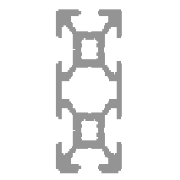
# Autodesk Inventor part: 3 842 992 891-0mm
Saved by Autodesk Inventor 2023.2 (Build 272271000, 271)
## iProperties
RuleStatus: InUse
Created: 2023-01-25
Part Number: 3 842 992 891-0mm
Material: Aluminum-6061
Description: PROFILE 20x40
Document SubType Name: Modeling
Designer: dmargari
Manufacturer: GENERIC
Standards Organization: ISO
Language: en-US
Size Designation: 300
Categories: <MemberInstance><Categories><Category DisplayName="Structural Shapes" InternalName="089c4875-fa83-4c05-b084-43b9cc11f5ed" Mnemonic="GRDR"><CategoryParameter DisplayName="Mass per Length Unit" InternalName="0bb95a10-148f-4027-a459-38d7b056702a" Mnemonic="shpmass"/><CategoryParameter DisplayName="Section Area" InternalName="1ff91680-64b0-4202-b9a3-7fd3f94bba3b" Mnemonic="secarea"/><CategoryParameter DisplayName="Radius of Gyration (x)" InternalName="25778675-03e9-40c1-b6a8-4a9ed693320d" Mnemonic="gyrradx"/><CategoryParameter DisplayName="Torsional Rigidity Modulus" InternalName="26c1ec35-5026-4c63-ad0a-751cf684a536" Mnemonic="torrigmod"/><CategoryParameter DisplayName="Distance of the Center of Gravity X-X" InternalName="26c9bdb8-9c79-4b4f-a92e-8e197583c9c4" Mnemonic="grcendistX"/><CategoryParameter DisplayName="Legacy Member ID" InternalName="340afe4f-75d7-48d3-ab7d-943f3c3da468" Mnemonic="LegacyMemberID"/><CategoryParameter DisplayName="Base Length" InternalName="42e34263-8f20-4d0e-ad48-bf1385b87c24" Mnemonic="shplen"/><CategoryParameter DisplayName="Moment of Inertia (y)" InternalName="4b9f58ea-bced-460e-81ea-3d29ca5a49e3" Mnemonic="inermomy"/><CategoryParameter DisplayName="Moment of Inertia (x)" InternalName="4cd780bc-73d7-43ac-917a-579e5cbd684d" Mnemonic="inermomx"/><CategoryParameter DisplayName="Custom Base Point" InternalName="4f1d1b73-316d-484b-a3df-9cbabb16eb77" Mnemonic="shpBasePoint"/><CategoryParameter DisplayName="Shape Height" InternalName="50274e7d-5ac0-4796-92cb-c59e54983c67" Mnemonic="shpheig"/><CategoryParameter DisplayName="Section Module (y)" InternalName="59eaa5e9-d227-48dc-b6c1-6920f96e0f95" Mnemonic="secmody"/><CategoryParameter DisplayName="Section Designation" InternalName="5a64d034-428d-49c8-ba32-7619764de20f" Mnemonic="shpdes"/><CategoryParameter DisplayName="Section Module (x)" InternalName="72cfad18-cf51-4ed4-aaa7-c6b224f8419f" Mnemonic="secmodx"/><CategoryParameter DisplayName="Torsional Section Modulus" InternalName="7c55a8dc-8844-49f9-a867-cc677b30ec9a" Mnemonic="torsecmod"/><CategoryParameter DisplayName="Shape Width" InternalName="7c717d54-a18f-4666-b4d4-573cce22c62c" Mnemonic="shpwdth"/><CategoryParameter DisplayName="Second Shape Thickness" InternalName="9251a8e1-85fd-4e47-af99-afdb762317d9" Mnemonic="shpthick2"/><CategoryParameter DisplayName="FG Authored" InternalName="9c666724-f362-4ea7-ac62-f6a007de5c69" Mnemonic="shpFGAuto"/><CategoryParameter DisplayName="Distance of the Center of Gravity Y-Y" InternalName="bcc4fb17-7af4-436a-8f8c-d0aa3b0248c5" Mnemonic="grcendistY"/><CategoryParameter DisplayName="Radius of Gyration (y)" InternalName="bfa18ebe-1636-4dbe-8d42-b263e0b73184" Mnemonic="gyrrady"/><CategoryParameter DisplayName="Shape Thickness" InternalName="d109cf76-8eb4-42fc-9800-4409734adc67" Mnemonic="shpthick"/><CategoryParameter DisplayName="Coefficient of Shear Displacement" InternalName="de4c90c6-aaa8-468f-a335-6737b311b5d3" Mnemonic="shdispc"/><Category DisplayName="Other" InternalName="f02205ff-2390-476f-921c-0b3185f88e84" Mnemonic="OTHSHP"><CategoryParameter DisplayName="Moment of Inertia (y)" InternalName="044c654e-f649-48ac-84cc-650a29ae31ca" Mnemonic="inermomy"/><CategoryParameter DisplayName="Shape Thickness" InternalName="12b1a788-9233-48fd-a933-2df8ff42b15f" Mnemonic="shpthick"/><CategoryParameter DisplayName="Mass per Length Unit" InternalName="2fd289d6-9394-4d2d-97e6-6659d7d4551d" Mnemonic="shpmass"/><CategoryParameter DisplayName="Radius of Gyration (y)" InternalName="743e1dfe-1bba-408b-b985-cf752b207386" Mnemonic="gyrrady"/><CategoryParameter DisplayName="Section Module (y)" InternalName="88b8bff9-a616-4028-93d5-ed4f79680d13" Mnemonic="secmody"/><CategoryParameter DisplayName="Section Area" InternalName="c46ecdf8-b6eb-4db9-8b25-30258930c1e3" Mnemonic="secarea"/><CategoryParameter DisplayName="Section Module (x)" InternalName="cac70804-9d39-43bb-be17-56ea1f39a6c2" Mnemonic="secmodx"/><CategoryParameter DisplayName="Moment of Inertia (x)" InternalName="ec6737bc-264f-43ed-b0bd-f6d410c2718d" Mnemonic="inermomx"/><CategoryParameter DisplayName="Radius of Gyration (x)" InternalName="ee72c61e-565e-4fd6-b448-66e1e1abcb7e" Mnemonic="gyrradx"/></Category></Category><Category DisplayName="DataType" InternalName="23b78d0f-2648-40c6-8793-ca6db495c9e8" Mnemonic="DATATYPE"><CategoryParameter DisplayName="DisplayName" InternalName="05415f3d-3907-474b-a020-eb9d644f4cf3" Mnemonic="DISPLAYNAME"/><CategoryParameter DisplayName="Standard" InternalName="0c0a119c-1e12-4c84-803f-101930972f5e" Mnemonic="STANDARD"/><CategoryParameter DisplayName="Description" InternalName="13903e3d-64b1-4950-80da-f627842ea37f" Mnemonic="DESCRIPTION"/><CategoryParameter DisplayName="Designation" InternalName="2675968c-4ce5-49e0-a4f5-552d29089031" Mnemonic="DESIGNATION"/><CategoryParameter DisplayName="Default Row" InternalName="2af9ec52-faaa-4026-b378-f9fa4afca842" Mnemonic="DEFAULTROW"/><CategoryParameter DisplayName="Folder Name" InternalName="3f06958e-8713-4116-9be7-ed6184ecc97b" Mnemonic="FOLDERNAME"/><CategoryParameter DisplayName="Revision Guid" InternalName="45a75005-10b1-4dfc-8d6d-dfe629f0b93c" Mnemonic="REVISIONGUID"/><CategoryParameter DisplayName="FileName" InternalName="8b46a4cc-9585-4fed-90c3-899f57e09a73" Mnemonic="FILENAME"/><CategoryParameter DisplayName="StdsOrg" InternalName="8f5914e1-4693-403f-8ab5-d37768198c9d" Mnemonic="STDSORG"/><CategoryParameter DisplayName="Family Version" InternalName="914462f6-6e19-4b14-ba84-155b9680b1d0" Mnemonic="FAMILYREVISION"/><CategoryParameter DisplayName="Standard Revision" InternalName="91d5a463-65c2-4fde-b823-3b7fea5e8e17" Mnemonic="STANDARDREVISION"/><CategoryParameter DisplayName="Member Revision" InternalName="a65d44b9-392f-4f4f-857b-e4b3d54996fe" Mnemonic="MEMBERREVISION"/><CategoryParameter DisplayName="ClipFormat" InternalName="bc51e27b-3422-4e78-93ef-cec197ddf230" Mnemonic="CLIPFORMAT"/><CategoryParameter DisplayName="Manufacturer" InternalName="cd6c7a72-a28a-4e50-99a9-2c7f4e13e5ad" Mnemonic="MANUFACTURER"/><CategoryParameter DisplayName="InternalName" InternalName="cf1d0246-76d9-4b4a-8305-fa0409afb5c1" Mnemonic="INTERNALNAME"/><CategoryParameter DisplayName="IsMetric" InternalName="e2385c5b-1ea4-4823-96a8-8de651266ec3" Mnemonic="ISMETRIC"/><Category DisplayName="Part" InternalName="c0e0b642-3bcb-4cc8-9e80-f96d35c4afa4" Mnemonic="PART"><CategoryParameter DisplayName="Part Number" InternalName="016b6077-bfbe-49bd-92c9-d8d59c39c941" Mnemonic="PARTNUMBER"/><CategoryParameter DisplayName="Stock Number" InternalName="4dba7c1c-e26c-444e-836c-b08b433409a8" Mnemonic="STOCKNUMBER"/><CategoryParameter DisplayName="Material Key" InternalName="5c9a8adb-dd2b-4535-b97f-0a94a95fe41f" Mnemonic="MATERIALKEY"/><CategoryParameter DisplayName="Material" InternalName="818a152a-d3c3-49ca-80ee-df7d91421b8e" Mnemonic="MATERIAL"/></Category></Category></Categories><FamilyTemplate Id="20x40"><FamilyTemplateParameters><FamilyTemplateParameter ObjectType="kModelParameterObject" ValueType="xs:double" Id="12" ObjectReferenceKey="Length"/><FamilyTemplateParameter ObjectType="kPartComponentDefinitionObject" ValueType="xs:string" Id="23" SubObjectId="Material"/><FamilyTemplateParameter ObjectType="kPropertyObject" ValueType="xs:string" Id="26" ObjectReferenceKey="{32853F0F-3444-11d1-9E93-0060B03C1CA6}" SubObjectId="5"/><FamilyTemplateParameter ObjectType="kPropertyObject" ValueType="xs:string" Id="27" ObjectReferenceKey="{32853F0F-3444-11d1-9E93-0060B03C1CA6}" SubObjectId="52"/></FamilyTemplateParameters></FamilyTemplate><CategoryParameterMap><ParamToTemplateMap><ParamToTemplate CategoryParameter="//CategoryParameter[@InternalName='cf1d0246-76d9-4b4a-8305-fa0409afb5c1']" ConstantValue="b55e8ed9-29f0-457f-be10-b8c2b92fdd42"/><ParamToTemplate CategoryParameter="//CategoryParameter[@InternalName='45a75005-10b1-4dfc-8d6d-dfe629f0b93c']" ConstantValue="8c683705-cc53-472d-bb0d-51e7db6332bf"/><ParamToTemplate CategoryParameter="//CategoryParameter[@InternalName='3f06958e-8713-4116-9be7-ed6184ecc97b']" ConstantValue="20x40"/><ParamToTemplate CategoryParameter="//CategoryParameter[@InternalName='8f5914e1-4693-403f-8ab5-d37768198c9d']" ConstantValue="ISO"/><ParamToTemplate CategoryParameter="//CategoryParameter[@InternalName='0c0a119c-1e12-4c84-803f-101930972f5e']" TemplateParameter="18"/><ParamToTemplate CategoryParameter="//CategoryParameter[@InternalName='91d5a463-65c2-4fde-b823-3b7fea5e8e17']" TemplateParameter="19"/><ParamToTemplate CategoryParameter="//CategoryParameter[@InternalName='cd6c7a72-a28a-4e50-99a9-2c7f4e13e5ad']" ConstantValue="GENERIC"/><ParamToTemplate CategoryParameter="//CategoryParameter[@InternalName='13903e3d-64b1-4950-80da-f627842ea37f']" ConstantValue="PROFILE 20x40"/><ParamToTemplate CategoryParameter="//CategoryParameter[@InternalName='05415f3d-3907-474b-a020-eb9d644f4cf3']" ConstantValue="20x40"/><ParamToTemplate CategoryParameter="//CategoryParameter[@InternalName='914462f6-6e19-4b14-ba84-155b9680b1d0']" ConstantValue="11"/><ParamToTemplate CategoryParameter="//CategoryParameter[@InternalName='bc51e27b-3422-4e78-93ef-cec197ddf230']" ConstantValue="CF_INVENTOR.STDPARTS"/><ParamToTemplate CategoryParameter="//CategoryParameter[@InternalName='e2385c5b-1ea4-4823-96a8-8de651266ec3']" ConstantValue="true"/><ParamToTemplate CategoryParameter="//CategoryParameter[@InternalName='2af9ec52-faaa-4026-b378-f9fa4afca842']" ConstantValue="1"/><ParamToTemplate CategoryParameter="//CategoryParameter[@InternalName='9c666724-f362-4ea7-ac62-f6a007de5c69']" ConstantValue="1"/><ParamToTemplate CategoryParameter="//CategoryParameter[@InternalName='8b46a4cc-9585-4fed-90c3-899f57e09a73']" ConstantValue="300"/><ParamToTemplate CategoryParameter="//CategoryParameter[@InternalName='a65d44b9-392f-4f4f-857b-e4b3d54996fe']" ConstantValue="6f428d9a-a522-4f2d-9c06-86253ee4d95b"/><ParamToTemplate CategoryParameter="//CategoryParameter[@InternalName='a65d44b9-392f-4f4f-857b-e4b3d54996fe']" ConstantValue="6f428d9a-a522-4f2d-9c06-86253ee4d95b"/><ParamToTemplate CategoryParameter="//CategoryParameter[@InternalName='2675968c-4ce5-49e0-a4f5-552d29089031']" TemplateParameter="27"/><ParamToTemplate CategoryParameter="//CategoryParameter[@InternalName='42e34263-8f20-4d0e-ad48-bf1385b87c24']" TemplateParameter="12"/><ParamToTemplate CategoryParameter="//CategoryParameter[@InternalName='818a152a-d3c3-49ca-80ee-df7d91421b8e']" TemplateParameter="23"/><ParamToTemplate CategoryParameter="//CategoryParameter[@InternalName='016b6077-bfbe-49bd-92c9-d8d59c39c941']" TemplateParameter="26"/></ParamToTemplateMap></CategoryParameterMap></MemberInstance>
Stock Number: 3 842 992 891
Mass: 1.55822 g
Surface Area: 12.24 cm^2
Volume: 0.57499 cm^3
Density: 2.71 g/cm^3
Appearance: Aluminum - Flat-1
IsCustomPart: 1
G_L: 300.000 mm
Author: dmargari
Autodesk Inventor part; units mm, degrees
(part 1 of 2)
ref_plane "YZ Plane" through (0, 0, 0) normal (1, 0, 0) x (0, 1, 0)
ref_plane "XZ Plane" through (0, 0, 0) normal (0, 1, 0) x (-1, 0, 0)
sketch "20x40" plane through (0, 0, 0) normal (0, 0, 1) x (1, 0, 0)
  line L0 (125.1239, 22.9032) -> (127.4025, 22.9032)
  arc A0 (127.5025, 22.8764) -> (127.4025, 22.9032) centre (127.4025, 22.7032) ccw
  line L1 (127.5025, 22.8764) -> (128.2563, 22.4412)
  arc A1 (128.2563, 22.4412) -> (128.4563, 22.4412) centre (128.3563, 22.6144) ccw
  line L2 (128.4563, 22.4412) -> (129.2101, 22.8764)
  arc A2 (129.3101, 22.9032) -> (129.2101, 22.8764) centre (129.3101, 22.7032) ccw
  line L3 (129.3101, 22.9032) -> (131.5887, 22.9032)
  arc A3 (131.5887, 22.9032) -> (131.9423, 23.0497) centre (131.5887, 23.4032) ccw
  line L4 (131.9423, 23.0497) -> (134.6492, 25.7567)
  arc A4 (135.0028, 25.9031) -> (134.6492, 25.7567) centre (135.0028, 25.4031) ccw
  line L5 (135.0028, 25.9031) -> (136.3563, 25.9031)
  arc A5 (136.3563, 25.9031) -> (136.8563, 26.4031) centre (136.3563, 26.4031) ccw
  line L6 (136.8563, 26.4031) -> (136.8563, 30.4031)
  arc A6 (136.8563, 30.4031) -> (136.3563, 30.9031) centre (136.3563, 30.4031) ccw
  line L7 (136.3563, 30.9031) -> (135.0028, 30.9031)
  arc A7 (134.6492, 31.0496) -> (135.0028, 30.9031) centre (135.0028, 31.4031) ccw
  line L8 (134.6492, 31.0496) -> (131.9421, 33.7567)
  arc A8 (131.9421, 33.7567) -> (131.5886, 33.9031) centre (131.5886, 33.4031) ccw
  line L9 (131.5886, 33.9031) -> (129.3099, 33.9031)
  arc A9 (129.2099, 33.9299) -> (129.3099, 33.9031) centre (129.3099, 34.1031) ccw
  line L10 (129.2099, 33.9299) -> (128.4563, 34.365)
  arc A10 (128.4563, 34.365) -> (128.2563, 34.365) centre (128.3563, 34.1918) ccw
  line L11 (128.2563, 34.365) -> (127.5027, 33.9299)
  arc A11 (134.2099, 45.3173) -> (134.3563, 45.6709) centre (133.8563, 45.6709) ccw
  line L12 (134.3563, 46.4031) -> (134.3563, 45.6709)
  arc A12 (134.3563, 46.4031) -> (133.8563, 46.9031) centre (133.8563, 46.4031) ccw
  line L13 (131.8563, 46.9031) -> (133.8563, 46.9031)
  arc A13 (131.3563, 47.4031) -> (131.8563, 46.9031) centre (131.8563, 47.4031) ccw
  line L14 (131.3563, 47.7031) -> (131.3563, 47.4031)
  arc A14 (131.5563, 47.9031) -> (131.3563, 47.7031) centre (131.5563, 47.7031) ccw
  line L15 (131.6563, 47.9031) -> (131.5563, 47.9031)
  arc A15 (131.6563, 47.9031) -> (131.8563, 48.1031) centre (131.6563, 48.1031) ccw
  line L16 (131.8563, 48.2031) -> (131.8563, 48.1031)
  arc A16 (132.0563, 48.4031) -> (131.8563, 48.2031) centre (132.0563, 48.2031) ccw
  line L17 (136.8563, 48.4031) -> (132.0563, 48.4031)
  arc A17 (138.3563, 46.9031) -> (136.8563, 48.4031) centre (136.8563, 46.9031) ccw
  line L18 (138.3563, 42.1031) -> (138.3563, 46.9031)
  arc A18 (138.1563, 41.9031) -> (138.3563, 42.1031) centre (138.1563, 42.1031) ccw
  line L19 (138.0563, 41.9031) -> (138.1563, 41.9031)
  arc A19 (138.0563, 41.9031) -> (137.8563, 41.7031) centre (138.0563, 41.7031) ccw
  line L20 (137.8563, 41.6031) -> (137.8563, 41.7031)
  arc A20 (137.6563, 41.4031) -> (137.8563, 41.6031) centre (137.6563, 41.6031) ccw
  line L21 (137.3563, 41.4031) -> (137.6563, 41.4031)
  arc A21 (136.8563, 41.9031) -> (137.3563, 41.4031) centre (137.3563, 41.9031) ccw
  line L22 (136.8563, 43.9031) -> (136.8563, 41.9031)
  arc A22 (136.8563, 43.9031) -> (136.3563, 44.4031) centre (136.3563, 43.9031) ccw
  line L23 (135.6241, 44.4031) -> (136.3563, 44.4031)
  arc A23 (135.6241, 44.4031) -> (135.2705, 44.2567) centre (135.6241, 43.9031) ccw
  line L24 (133.0028, 41.9889) -> (135.2705, 44.2567)
  arc A24 (133.0028, 41.9889) -> (132.8563, 41.6353) centre (133.3563, 41.6353) ccw
  line L25 (132.8563, 39.3567) -> (132.8563, 41.6353)
  arc A25 (132.8295, 39.2567) -> (132.8563, 39.3567) centre (132.6563, 39.3567) ccw
  line L26 (132.3944, 38.5031) -> (132.8295, 39.2567)
  arc A26 (132.3944, 38.5031) -> (132.3944, 38.3031) centre (132.5676, 38.4031) ccw
  line L27 (132.8295, 37.5495) -> (132.3944, 38.3031)
  arc A27 (132.8563, 37.4495) -> (132.8295, 37.5495) centre (132.6563, 37.4495) ccw
  line L28 (132.8563, 35.1709) -> (132.8563, 37.4495)
  arc A28 (132.8563, 35.1709) -> (133.0028, 34.8173) centre (133.3563, 35.1709) ccw
  line L29 (135.2705, 32.5496) -> (133.0028, 34.8173)
  arc A29 (135.2705, 32.5496) -> (135.6241, 32.4031) centre (135.6241, 32.9031) ccw
  line L30 (136.3563, 32.4031) -> (135.6241, 32.4031)
  arc A30 (136.3563, 32.4031) -> (136.8563, 32.9031) centre (136.3563, 32.9031) ccw
  line L31 (136.8563, 34.9031) -> (136.8563, 32.9031)
  arc A31 (137.3563, 35.4031) -> (136.8563, 34.9031) centre (137.3563, 34.9031) ccw
  line L32 (137.6563, 35.4031) -> (137.3563, 35.4031)
  arc A32 (137.8563, 35.2031) -> (137.6563, 35.4031) centre (137.6563, 35.2031) ccw
  line L33 (137.8563, 35.1031) -> (137.8563, 35.2031)
  arc A33 (137.8563, 35.1031) -> (138.0563, 34.9031) centre (138.0563, 35.1031) ccw
  line L34 (138.1563, 34.9031) -> (138.0563, 34.9031)
  arc A34 (138.3563, 34.7031) -> (138.1563, 34.9031) centre (138.1563, 34.7031) ccw
  line L35 (138.3563, 22.0531) -> (138.3563, 34.7031)
  arc A35 (138.1563, 21.8531) -> (138.3563, 22.0531) centre (138.1563, 22.0531) ccw
  line L36 (138.0563, 21.8531) -> (138.1563, 21.8531)
  arc A36 (138.0563, 21.8531) -> (137.8563, 21.6531) centre (138.0563, 21.6531) ccw
  line L37 (137.8563, 21.5531) -> (137.8563, 21.6531)
  arc A37 (137.6563, 21.3531) -> (137.8563, 21.5531) centre (137.6563, 21.5531) ccw
  line L38 (137.3563, 21.3531) -> (137.6563, 21.3531)
  arc A38 (136.8563, 21.8531) -> (137.3563, 21.3531) centre (137.3563, 21.8531) ccw
  line L39 (136.8563, 23.9031) -> (136.8563, 21.8531)
  arc A39 (136.8563, 23.9031) -> (136.3563, 24.4031) centre (136.3563, 23.9031) ccw
  line L40 (135.6241, 24.4031) -> (136.3563, 24.4031)
  arc A40 (135.6241, 24.4031) -> (135.2705, 24.2567) centre (135.6241, 23.9031) ccw
  line L41 (133.0028, 21.9889) -> (135.2705, 24.2567)
  arc A41 (133.0028, 21.9889) -> (132.8563, 21.6353) centre (133.3563, 21.6353) ccw
  line L42 (132.8563, 19.3567) -> (132.8563, 21.6353)
  arc A42 (132.8295, 19.2567) -> (132.8563, 19.3567) centre (132.6563, 19.3567) ccw
  line L43 (132.3944, 18.5031) -> (132.8295, 19.2567)
  arc A43 (132.3944, 18.5031) -> (132.3944, 18.3031) centre (132.5676, 18.4031) ccw
  line L44 (132.8295, 17.5495) -> (132.3944, 18.3031)
  arc A44 (132.8563, 17.4495) -> (132.8295, 17.5495) centre (132.6563, 17.4495) ccw
  line L45 (132.8563, 15.1709) -> (132.8563, 17.4495)
  arc A45 (132.8563, 15.1709) -> (133.0028, 14.8173) centre (133.3563, 15.1709) ccw
  line L46 (135.2705, 12.5496) -> (133.0028, 14.8173)
  arc A46 (135.2705, 12.5496) -> (135.6241, 12.4031) centre (135.6241, 12.9031) ccw
  line L47 (136.3563, 12.4031) -> (135.6241, 12.4031)
  arc A47 (136.3563, 12.4031) -> (136.8563, 12.9031) centre (136.3563, 12.9031) ccw
  line L48 (136.8563, 14.8531) -> (136.8563, 12.9031)
  arc A48 (137.3563, 15.3531) -> (136.8563, 14.8531) centre (137.3563, 14.8531) ccw
  line L49 (137.6563, 15.3531) -> (137.3563, 15.3531)
  arc A49 (137.8563, 15.1531) -> (137.6563, 15.3531) centre (137.6563, 15.1531) ccw
  line L50 (137.8563, 15.0531) -> (137.8563, 15.1531)
  arc A50 (137.8563, 15.0531) -> (138.0563, 14.8531) centre (138.0563, 15.0531) ccw
  line L51 (138.1563, 14.8531) -> (138.0563, 14.8531)
  arc A51 (138.3563, 14.6531) -> (138.1563, 14.8531) centre (138.1563, 14.6531) ccw
  arc A52 (127.4027, 33.9031) -> (127.5027, 33.9299) centre (127.4027, 34.1031) ccw
  line L52 (127.4027, 33.9031) -> (125.1241, 33.9031)
  arc A53 (125.1241, 33.9031) -> (124.7705, 33.7567) centre (125.1241, 33.4031) ccw
  line L53 (124.7705, 33.7567) -> (122.0634, 31.0496)
  arc A54 (121.7099, 30.9031) -> (122.0634, 31.0496) centre (121.7099, 31.4031) ccw
  line L54 (121.7099, 30.9031) -> (120.3563, 30.9031)
  arc A55 (120.3563, 30.9031) -> (119.8563, 30.4031) centre (120.3563, 30.4031) ccw
  line L55 (119.8563, 30.4031) -> (119.8563, 26.4031)
  arc A56 (119.8563, 26.4031) -> (120.3563, 25.9031) centre (120.3563, 26.4031) ccw
  line L56 (120.3563, 25.9031) -> (121.7099, 25.9031)
  arc A57 (122.0634, 25.7567) -> (121.7099, 25.9031) centre (121.7099, 25.4031) ccw
  line L57 (122.0634, 25.7567) -> (124.7703, 23.0497)
  arc A58 (124.7703, 23.0497) -> (125.1239, 22.9032) centre (125.1239, 23.4032) ccw
  arc A59 (118.3563, 9.9031) -> (119.8563, 8.4031) centre (119.8563, 9.9031) ccw
  line L58 (118.3563, 14.6531) -> (118.3563, 9.9031)
  arc A60 (118.5563, 14.8531) -> (118.3563, 14.6531) centre (118.5563, 14.6531) ccw
  line L59 (118.6563, 14.8531) -> (118.5563, 14.8531)
  arc A61 (118.6563, 14.8531) -> (118.8563, 15.0531) centre (118.6563, 15.0531) ccw
  line L60 (118.8563, 15.1531) -> (118.8563, 15.0531)
  arc A62 (119.0563, 15.3531) -> (118.8563, 15.1531) centre (119.0563, 15.1531) ccw
  line L61 (119.3563, 15.3531) -> (119.0563, 15.3531)
  arc A63 (119.8563, 14.8531) -> (119.3563, 15.3531) centre (119.3563, 14.8531) ccw
  line L62 (119.8563, 12.9031) -> (119.8563, 14.8531)
  arc A64 (119.8563, 12.9031) -> (120.3563, 12.4031) centre (120.3563, 12.9031) ccw
  line L63 (121.0885, 12.4031) -> (120.3563, 12.4031)
  arc A65 (121.0885, 12.4031) -> (121.4421, 12.5496) centre (121.0885, 12.9031) ccw
  line L64 (123.7099, 14.8173) -> (121.4421, 12.5496)
  arc A66 (123.7099, 14.8173) -> (123.8563, 15.1709) centre (123.3563, 15.1709) ccw
  line L65 (123.8563, 17.4495) -> (123.8563, 15.1709)
  arc A67 (123.8831, 17.5495) -> (123.8563, 17.4495) centre (124.0563, 17.4495) ccw
  line L66 (124.3182, 18.3031) -> (123.8831, 17.5495)
  arc A68 (124.3182, 18.3031) -> (124.3182, 18.5031) centre (124.145, 18.4031) ccw
  line L67 (123.8831, 19.2567) -> (124.3182, 18.5031)
  arc A69 (123.8563, 19.3567) -> (123.8831, 19.2567) centre (124.0563, 19.3567) ccw
  line L68 (123.8563, 21.6353) -> (123.8563, 19.3567)
  arc A70 (123.8563, 21.6353) -> (123.7099, 21.9889) centre (123.3563, 21.6353) ccw
  line L69 (121.4421, 24.2567) -> (123.7099, 21.9889)
  arc A71 (121.4421, 24.2567) -> (121.0886, 24.4031) centre (121.0886, 23.9031) ccw
  line L70 (120.3563, 24.4031) -> (121.0886, 24.4031)
  arc A72 (120.3563, 24.4031) -> (119.8563, 23.9031) centre (120.3563, 23.9031) ccw
  line L71 (119.8563, 21.8531) -> (119.8563, 23.9031)
  arc A73 (119.3563, 21.3531) -> (119.8563, 21.8531) centre (119.3563, 21.8531) ccw
  line L72 (119.0563, 21.3531) -> (119.3563, 21.3531)
  arc A74 (118.8563, 21.5531) -> (119.0563, 21.3531) centre (119.0563, 21.5531) ccw
  line L73 (118.8563, 21.6531) -> (118.8563, 21.5531)
  arc A75 (118.8563, 21.6531) -> (118.6563, 21.8531) centre (118.6563, 21.6531) ccw
  line L74 (118.5563, 21.8531) -> (118.6563, 21.8531)
  arc A76 (118.3563, 22.0531) -> (118.5563, 21.8531) centre (118.5563, 22.0531) ccw
  line L75 (118.3563, 34.7031) -> (118.3563, 22.0531)
  arc A77 (118.5563, 34.9031) -> (118.3563, 34.7031) centre (118.5563, 34.7031) ccw
  line L76 (118.6563, 34.9031) -> (118.5563, 34.9031)
  arc A78 (118.6563, 34.9031) -> (118.8563, 35.1031) centre (118.6563, 35.1031) ccw
  line L77 (118.8563, 35.2031) -> (118.8563, 35.1031)
  arc A79 (119.0563, 35.4031) -> (118.8563, 35.2031) centre (119.0563, 35.2031) ccw
  line L78 (119.3563, 35.4031) -> (119.0563, 35.4031)
  arc A80 (119.8563, 34.9031) -> (119.3563, 35.4031) centre (119.3563, 34.9031) ccw
  line L79 (119.8563, 32.9531) -> (119.8563, 34.9031)
  arc A81 (119.8563, 32.9531) -> (120.3563, 32.4531) centre (120.3563, 32.9531) ccw
  line L80 (121.1386, 32.4531) -> (120.3563, 32.4531)
  arc A82 (121.1386, 32.4531) -> (121.4921, 32.5996) centre (121.1386, 32.9531) ccw
  line L81 (123.7099, 34.8173) -> (121.4921, 32.5996)
  arc A83 (123.7099, 34.8173) -> (123.8563, 35.1709) centre (123.3563, 35.1709) ccw
  line L82 (123.8563, 37.4495) -> (123.8563, 35.1709)
  arc A84 (123.8831, 37.5495) -> (123.8563, 37.4495) centre (124.0563, 37.4495) ccw
  line L83 (124.3182, 38.3031) -> (123.8831, 37.5495)
  arc A85 (124.3182, 38.3031) -> (124.3182, 38.5031) centre (124.145, 38.4031) ccw
  line L84 (123.8831, 39.2567) -> (124.3182, 38.5031)
  arc A86 (123.8563, 39.3567) -> (123.8831, 39.2567) centre (124.0563, 39.3567) ccw
  line L85 (123.8563, 41.6353) -> (123.8563, 39.3567)
  arc A87 (123.8563, 41.6353) -> (123.7099, 41.9889) centre (123.3563, 41.6353) ccw
  line L86 (121.3921, 44.3067) -> (123.7099, 41.9889)
  arc A88 (121.3921, 44.3067) -> (121.0386, 44.4531) centre (121.0386, 43.9531) ccw
  line L87 (120.3563, 44.4531) -> (121.0386, 44.4531)
  arc A89 (120.3563, 44.4531) -> (119.8563, 43.9531) centre (120.3563, 43.9531) ccw
  line L88 (119.8563, 41.9031) -> (119.8563, 43.9531)
  arc A90 (119.3563, 41.4031) -> (119.8563, 41.9031) centre (119.3563, 41.9031) ccw
  line L89 (119.0563, 41.4031) -> (119.3563, 41.4031)
  arc A91 (118.8563, 41.6031) -> (119.0563, 41.4031) centre (119.0563, 41.6031) ccw
  line L90 (118.8563, 41.7031) -> (118.8563, 41.6031)
  arc A92 (118.8563, 41.7031) -> (118.6563, 41.9031) centre (118.6563, 41.7031) ccw
  line L91 (118.5563, 41.9031) -> (118.6563, 41.9031)
  arc A93 (118.3563, 42.1031) -> (118.5563, 41.9031) centre (118.5563, 42.1031) ccw
  line L92 (118.3563, 46.9031) -> (118.3563, 42.1031)
  arc A94 (119.8563, 48.4031) -> (118.3563, 46.9031) centre (119.8563, 46.9031) ccw
  line L93 (124.6563, 48.4031) -> (119.8563, 48.4031)
  arc A95 (124.8563, 48.2031) -> (124.6563, 48.4031) centre (124.6563, 48.2031) ccw
  line L94 (124.8563, 48.1031) -> (124.8563, 48.2031)
  arc A96 (124.8563, 48.1031) -> (125.0563, 47.9031) centre (125.0563, 48.1031) ccw
  line L95 (125.1563, 47.9031) -> (125.0563, 47.9031)
  arc A97 (125.3563, 47.7031) -> (125.1563, 47.9031) centre (125.1563, 47.7031) ccw
  line L96 (125.3563, 47.4031) -> (125.3563, 47.7031)
  arc A98 (124.8563, 46.9031) -> (125.3563, 47.4031) centre (124.8563, 47.4031) ccw
  line L97 (122.8563, 46.9031) -> (124.8563, 46.9031)
  arc A99 (122.8563, 46.9031) -> (122.3563, 46.4031) centre (122.8563, 46.4031) ccw
  line L98 (122.3563, 45.6709) -> (122.3563, 46.4031)
  arc A100 (122.3563, 45.6709) -> (122.5028, 45.3173) centre (122.8563, 45.6709) ccw
  line L99 (124.7704, 43.0496) -> (122.5028, 45.3173)
  arc A101 (124.7704, 43.0496) -> (125.124, 42.9032) centre (125.124, 43.4032) ccw
  line L100 (127.4026, 42.9032) -> (125.124, 42.9032)
  arc A102 (127.5026, 42.8764) -> (127.4026, 42.9032) centre (127.4026, 42.7032) ccw
  line L101 (128.2563, 42.4412) -> (127.5026, 42.8764)
  arc A103 (128.2563, 42.4412) -> (128.4563, 42.4412) centre (128.3563, 42.6144) ccw
  line L102 (129.21, 42.8764) -> (128.4563, 42.4412)
  arc A104 (129.31, 42.9032) -> (129.21, 42.8764) centre (129.31, 42.7032) ccw
  line L103 (131.5886, 42.9032) -> (129.31, 42.9032)
  arc A105 (131.5886, 42.9032) -> (131.9422, 43.0496) centre (131.5886, 43.4032) ccw
  line L104 (134.2099, 45.3173) -> (131.9422, 43.0496)
  arc A106 (137.8563, 15.1531) -> (137.6563, 15.3531) centre (137.6563, 15.1531) ccw
  arc A107 (138.3563, 14.6531) -> (138.1563, 14.8531) centre (138.1563, 14.6531) ccw
  arc A108 (137.8563, 15.0531) -> (138.0563, 14.8531) centre (138.0563, 15.0531) ccw
  arc A109 (137.3563, 15.3531) -> (136.8563, 14.8531) centre (137.3563, 14.8531) ccw
  arc A110 (138.0563, 21.8531) -> (137.8563, 21.6531) centre (138.0563, 21.6531) ccw
  arc A111 (138.1563, 21.8531) -> (138.3563, 22.0531) centre (138.1563, 22.0531) ccw
  arc A112 (137.6563, 21.3531) -> (137.8563, 21.5531) centre (137.6563, 21.5531) ccw
  arc A113 (136.8563, 21.8531) -> (137.3563, 21.3531) centre (137.3563, 21.8531) ccw
  arc A114 (118.8563, 21.6531) -> (118.6563, 21.8531) centre (118.6563, 21.6531) ccw
  arc A115 (118.3563, 22.0531) -> (118.5563, 21.8531) centre (118.5563, 22.0531) ccw
  arc A116 (118.8563, 21.5531) -> (119.0563, 21.3531) centre (119.0563, 21.5531) ccw
  arc A117 (119.3563, 21.3531) -> (119.8563, 21.8531) centre (119.3563, 21.8531) ccw
  arc A118 (118.6563, 14.8531) -> (118.8563, 15.0531) centre (118.6563, 15.0531) ccw
  arc A119 (118.5563, 14.8531) -> (118.3563, 14.6531) centre (118.5563, 14.6531) ccw
  arc A120 (119.0563, 15.3531) -> (118.8563, 15.1531) centre (119.0563, 15.1531) ccw
  arc A121 (119.8563, 14.8531) -> (119.3563, 15.3531) centre (119.3563, 14.8531) ccw
  arc A122 (125.1563, 8.9031) -> (125.3563, 9.1031) centre (125.1563, 9.1031) ccw
  arc A123 (124.6563, 8.4031) -> (124.8563, 8.6031) centre (124.6563, 8.6031) ccw
  arc A124 (125.0563, 8.9031) -> (124.8563, 8.7031) centre (125.0563, 8.7031) ccw
  arc A125 (125.3563, 9.4031) -> (124.8563, 9.9031) centre (124.8563, 9.4031) ccw
  arc A126 (131.8563, 8.7031) -> (131.6563, 8.9031) centre (131.6563, 8.7031) ccw
  arc A127 (131.8563, 8.6031) -> (132.0563, 8.4031) centre (132.0563, 8.6031) ccw
  arc A128 (131.3563, 9.1031) -> (131.5563, 8.9031) centre (131.5563, 9.1031) ccw
  arc A129 (131.8563, 9.9031) -> (131.3563, 9.4031) centre (131.8563, 9.4031) ccw
  arc A130 (118.8563, 41.7031) -> (118.6563, 41.9031) centre (118.6563, 41.7031) ccw
  arc A131 (118.3563, 42.1031) -> (118.5563, 41.9031) centre (118.5563, 42.1031) ccw
  arc A132 (118.8563, 41.6031) -> (119.0563, 41.4031) centre (119.0563, 41.6031) ccw
  arc A133 (119.3563, 41.4031) -> (119.8563, 41.9031) centre (119.3563, 41.9031) ccw
  arc A134 (118.6563, 34.9031) -> (118.8563, 35.1031) centre (118.6563, 35.1031) ccw
  arc A135 (118.5563, 34.9031) -> (118.3563, 34.7031) centre (118.5563, 34.7031) ccw
  arc A136 (119.0563, 35.4031) -> (118.8563, 35.2031) centre (119.0563, 35.2031) ccw
  arc A137 (119.8563, 34.9031) -> (119.3563, 35.4031) centre (119.3563, 34.9031) ccw
  arc A138 (137.8563, 35.2031) -> (137.6563, 35.4031) centre (137.6563, 35.2031) ccw
  arc A139 (138.3563, 34.7031) -> (138.1563, 34.9031) centre (138.1563, 34.7031) ccw
  arc A140 (137.8563, 35.1031) -> (138.0563, 34.9031) centre (138.0563, 35.1031) ccw
  arc A141 (137.3563, 35.4031) -> (136.8563, 34.9031) centre (137.3563, 34.9031) ccw
  arc A142 (138.0563, 41.9031) -> (137.8563, 41.7031) centre (138.0563, 41.7031) ccw
  arc A143 (138.1563, 41.9031) -> (138.3563, 42.1031) centre (138.1563, 42.1031) ccw
  arc A144 (137.6563, 41.4031) -> (137.8563, 41.6031) centre (137.6563, 41.6031) ccw
  arc A145 (136.8563, 41.9031) -> (137.3563, 41.4031) centre (137.3563, 41.9031) ccw
  arc A146 (125.3563, 47.7031) -> (125.1563, 47.9031) centre (125.1563, 47.7031) ccw
  arc A147 (124.8563, 48.2031) -> (124.6563, 48.4031) centre (124.6563, 48.2031) ccw
  arc A148 (124.8563, 48.1031) -> (125.0563, 47.9031) centre (125.0563, 48.1031) ccw
  arc A149 (124.8563, 46.9031) -> (125.3563, 47.4031) centre (124.8563, 47.4031) ccw
  arc A150 (131.5563, 47.9031) -> (131.3563, 47.7031) centre (131.5563, 47.7031) ccw
  arc A151 (132.0563, 48.4031) -> (131.8563, 48.2031) centre (132.0563, 48.2031) ccw
  arc A152 (131.6563, 47.9031) -> (131.8563, 48.1031) centre (131.6563, 48.1031) ccw
  arc A153 (131.3563, 47.4031) -> (131.8563, 46.9031) centre (131.8563, 47.4031) ccw
  arc A154 (130.8016, 37.1449) -> (130.8016, 39.6613) centre (128.3563, 38.4031) ccw
  arc A155 (127.0981, 35.9578) -> (129.6145, 35.9578) centre (128.3563, 38.4031) ccw
  arc A156 (125.911, 39.6613) -> (125.911, 37.1449) centre (128.3563, 38.4031) ccw
  arc A157 (130.2434, 35.4554) -> (131.304, 36.5161) centre (128.3563, 38.4031) ccw
  arc A158 (125.4086, 36.5161) -> (126.4693, 35.4554) centre (128.3563, 38.4031) ccw
  arc A159 (126.4693, 41.3508) -> (125.4086, 40.2902) centre (128.3563, 38.4031) ccw
  arc A160 (131.304, 40.2902) -> (130.2434, 41.3508) centre (128.3563, 38.4031) ccw
  arc A161 (132.3944, 38.5031) -> (132.3944, 38.3031) centre (132.5676, 38.4031) ccw
  arc A162 (132.8563, 37.4495) -> (132.8295, 37.5495) centre (132.6563, 37.4495) ccw
  arc A163 (132.8295, 39.2567) -> (132.8563, 39.3567) centre (132.6563, 39.3567) ccw
  arc A164 (135.2705, 32.5496) -> (135.6241, 32.4031) centre (135.6241, 32.9031) ccw
  arc A165 (132.8563, 35.1709) -> (133.0028, 34.8173) centre (133.3563, 35.1709) ccw
  arc A166 (133.0028, 41.9889) -> (132.8563, 41.6353) centre (133.3563, 41.6353) ccw
  arc A167 (135.6241, 44.4031) -> (135.2705, 44.2567) centre (135.6241, 43.9031) ccw
  arc A168 (128.4563, 34.365) -> (128.2563, 34.365) centre (128.3563, 34.1918) ccw
  arc A169 (127.4027, 33.9031) -> (127.5027, 33.9299) centre (127.4027, 34.1031) ccw
  line L105 (127.5025, 22.8764) -> (128.2563, 22.4412)
  line L106 (129.2101, 22.8764) -> (128.4563, 22.4412)
  line L107 (131.5887, 22.9032) -> (129.3101, 22.9032)
  line L108 (133.0028, 21.9889) -> (135.2705, 24.2567)
  line L109 (130.8016, 17.1449) -> (131.304, 16.5161)
  line L110 (135.6241, 24.4031) -> (136.3563, 24.4031)
  line L111 (135.6241, 12.4031) -> (136.3563, 12.4031)
  line L112 (132.8563, 21.6353) -> (132.8563, 19.3567)
  line L113 (132.8295, 19.2567) -> (132.3944, 18.5031)
  line L114 (132.8295, 17.5495) -> (132.3944, 18.3031)
  line L115 (132.8563, 15.1709) -> (132.8563, 17.4495)
  line L116 (133.0028, 14.8173) -> (135.2705, 12.5496)
  line L117 (131.9421, 13.7567) -> (134.2099, 11.4889)
  line L118 (127.0981, 15.9578) -> (126.4693, 15.4554)
  line L119 (125.911, 17.1449) -> (125.4086, 16.5161)
  line L120 (125.911, 19.6613) -> (125.4086, 20.2902)
  line L121 (127.0981, 20.8484) -> (126.4693, 21.3508)
  line L122 (129.6145, 20.8484) -> (130.2434, 21.3508)
  line L123 (130.8016, 19.6613) -> (131.304, 20.2902)
  line L124 (135.0028, 30.9031) -> (136.3563, 30.9031)
  line L125 (136.8563, 26.4031) -> (136.8563, 30.4031)
  line L126 (135.0028, 25.9031) -> (136.3563, 25.9031)
  line L127 (121.7099, 25.9031) -> (120.3563, 25.9031)
  line L128 (119.8563, 26.4031) -> (119.8563, 30.4031)
  line L129 (121.7099, 30.9031) -> (120.3563, 30.9031)
  arc A170 (130.2434, 15.4554) -> (131.304, 16.5161) centre (128.3563, 18.4031) ccw
  line L130 (131.304, 16.5161) -> (130.8016, 17.1449)
  arc A171 (130.8016, 17.1449) -> (130.8016, 19.6613) centre (128.3563, 18.4031) ccw
  line L131 (130.8016, 19.6613) -> (131.304, 20.2902)
  arc A172 (131.304, 20.2902) -> (130.2434, 21.3508) centre (128.3563, 18.4031) ccw
  line L132 (130.2434, 21.3508) -> (129.6145, 20.8484)
  arc A173 (129.6145, 20.8484) -> (127.0981, 20.8484) centre (128.3563, 18.4031) ccw
  line L133 (127.0981, 20.8484) -> (126.4693, 21.3508)
  arc A174 (126.4693, 21.3508) -> (125.4086, 20.2902) centre (128.3563, 18.4031) ccw
  line L134 (125.4086, 20.2902) -> (125.911, 19.6613)
  arc A175 (125.911, 19.6613) -> (125.911, 17.1449) centre (128.3563, 18.4031) ccw
  line L135 (125.911, 17.1449) -> (125.4086, 16.5161)
  arc A176 (125.4086, 16.5161) -> (126.4693, 15.4554) centre (128.3563, 18.4031) ccw
  line L136 (126.4693, 15.4554) -> (127.0981, 15.9578)
  arc A177 (127.0981, 15.9578) -> (129.6145, 15.9578) centre (128.3563, 18.4031) ccw
  line L137 (129.6145, 15.9578) -> (130.2434, 15.4554)
  arc A178 (131.304, 40.2902) -> (130.2434, 41.3508) centre (128.3563, 38.4031) ccw
  line L138 (130.2434, 41.3508) -> (129.6145, 40.8484)
  arc A179 (129.6145, 40.8484) -> (127.0981, 40.8484) centre (128.3563, 38.4031) ccw
  line L139 (127.0981, 40.8484) -> (126.4693, 41.3508)
  arc A180 (126.4693, 41.3508) -> (125.4086, 40.2902) centre (128.3563, 38.4031) ccw
  line L140 (125.4086, 40.2902) -> (125.911, 39.6613)
  arc A181 (125.911, 39.6613) -> (125.911, 37.1449) centre (128.3563, 38.4031) ccw
  line L141 (125.911, 37.1449) -> (125.4086, 36.5161)
  arc A182 (125.4086, 36.5161) -> (126.4693, 35.4554) centre (128.3563, 38.4031) ccw
  line L142 (126.4693, 35.4554) -> (127.0981, 35.9578)
  arc A183 (127.0981, 35.9578) -> (129.6145, 35.9578) centre (128.3563, 38.4031) ccw
  line L143 (129.6145, 35.9578) -> (130.2434, 35.4554)
  arc A184 (130.2434, 35.4554) -> (131.304, 36.5161) centre (128.3563, 38.4031) ccw
  line L144 (131.304, 36.5161) -> (130.8016, 37.1449)
  arc A185 (130.8016, 37.1449) -> (130.8016, 39.6613) centre (128.3563, 38.4031) ccw
  line L145 (130.8016, 39.6613) -> (131.304, 40.2902)
  line L146 (138.3563, 9.9031) -> (138.3563, 14.6531)
  arc A186 (136.8563, 8.4031) -> (138.3563, 9.9031) centre (136.8563, 9.9031) ccw
  line L147 (132.0563, 8.4031) -> (136.8563, 8.4031)
  arc A187 (131.8563, 8.6031) -> (132.0563, 8.4031) centre (132.0563, 8.6031) ccw
  line L148 (131.8563, 8.7031) -> (131.8563, 8.6031)
  arc A188 (131.8563, 8.7031) -> (131.6563, 8.9031) centre (131.6563, 8.7031) ccw
  line L149 (131.5563, 8.9031) -> (131.6563, 8.9031)
  arc A189 (131.3563, 9.1031) -> (131.5563, 8.9031) centre (131.5563, 9.1031) ccw
  line L150 (131.3563, 9.4031) -> (131.3563, 9.1031)
  arc A190 (131.8563, 9.9031) -> (131.3563, 9.4031) centre (131.8563, 9.4031) ccw
  line L151 (133.8563, 9.9031) -> (131.8563, 9.9031)
  arc A191 (133.8563, 9.9031) -> (134.3563, 10.4031) centre (133.8563, 10.4031) ccw
  line L152 (134.3563, 11.1353) -> (134.3563, 10.4031)
  arc A192 (134.3563, 11.1353) -> (134.2099, 11.4889) centre (133.8563, 11.1353) ccw
  line L153 (131.9421, 13.7567) -> (134.2099, 11.4889)
  arc A193 (131.9421, 13.7567) -> (131.5885, 13.9031) centre (131.5885, 13.4031) ccw
  line L154 (129.3099, 13.9031) -> (131.5885, 13.9031)
  arc A194 (129.2099, 13.9299) -> (129.3099, 13.9031) centre (129.3099, 14.1031) ccw
  line L155 (128.4563, 14.365) -> (129.2099, 13.9299)
  arc A195 (128.4563, 14.365) -> (128.2563, 14.365) centre (128.3563, 14.1918) ccw
  line L156 (127.5027, 13.9299) -> (128.2563, 14.365)
  arc A196 (127.4027, 13.9031) -> (127.5027, 13.9299) centre (127.4027, 14.1031) ccw
  line L157 (125.1241, 13.9031) -> (127.4027, 13.9031)
  arc A197 (125.1241, 13.9031) -> (124.7705, 13.7567) centre (125.1241, 13.4031) ccw
  line L158 (122.5028, 11.4889) -> (124.7705, 13.7567)
  arc A198 (122.5028, 11.4889) -> (122.3563, 11.1353) centre (122.8563, 11.1353) ccw
  line L159 (122.3563, 10.4031) -> (122.3563, 11.1353)
  arc A199 (122.3563, 10.4031) -> (122.8563, 9.9031) centre (122.8563, 10.4031) ccw
  line L160 (124.8563, 9.9031) -> (122.8563, 9.9031)
  arc A200 (125.3563, 9.4031) -> (124.8563, 9.9031) centre (124.8563, 9.4031) ccw
  line L161 (125.3563, 9.1031) -> (125.3563, 9.4031)
  arc A201 (125.1563, 8.9031) -> (125.3563, 9.1031) centre (125.1563, 9.1031) ccw
  line L162 (125.0563, 8.9031) -> (125.1563, 8.9031)
  arc A202 (125.0563, 8.9031) -> (124.8563, 8.7031) centre (125.0563, 8.7031) ccw
  line L163 (124.8563, 8.6031) -> (124.8563, 8.7031)
  arc A203 (124.6563, 8.4031) -> (124.8563, 8.6031) centre (124.6563, 8.6031) ccw
  line L164 (119.8563, 8.4031) -> (124.6563, 8.4031)
  line L165 (136.8563, 21.8531) -> (136.8563, 23.9031)
  line L166 (138.3563, 22.0531) -> (138.3563, 28.4031)
  line L167 (118.6563, 21.8531) -> (118.5563, 21.8531)
  line L168 (118.8563, 21.5531) -> (118.8563, 21.6531)
  line L169 (119.3563, 21.3531) -> (119.0563, 21.3531)
  line L170 (119.8563, 21.8531) -> (119.8563, 23.9031)
  line L171 (118.3563, 22.0531) -> (118.3563, 28.4031)
  line L172 (118.6563, 14.8531) -> (118.5563, 14.8531)
  line L173 (118.8563, 15.1531) -> (118.8563, 15.0531)
  line L174 (119.3563, 15.3531) -> (119.0563, 15.3531)
  line L175 (119.8563, 14.8531) -> (119.8563, 12.9031)
  line L176 (118.3563, 14.6531) -> (118.3563, 9.9031)
  line L177 (124.6563, 8.4031) -> (119.8563, 8.4031)
  line L178 (124.8563, 9.9031) -> (122.8563, 9.9031)
  line L179 (125.1563, 8.9031) -> (125.0563, 8.9031)
  line L180 (124.8563, 8.7031) -> (124.8563, 8.6031)
  line L181 (125.3563, 9.4031) -> (125.3563, 9.1031)
  line L182 (132.0563, 8.4031) -> (136.8563, 8.4031)
  line L183 (131.8563, 8.7031) -> (131.8563, 8.6031)
  line L184 (131.5563, 8.9031) -> (131.6563, 8.9031)
  line L185 (131.3563, 9.4031) -> (131.3563, 9.1031)
  line L186 (131.8563, 9.9031) -> (133.8563, 9.9031)
  line L187 (118.6563, 41.9031) -> (118.5563, 41.9031)
  line L188 (118.8563, 41.6031) -> (118.8563, 41.7031)
  line L189 (119.3563, 41.4031) -> (119.0563, 41.4031)
  line L190 (119.8563, 41.9031) -> (119.8563, 43.9531)
  line L191 (118.3563, 42.1031) -> (118.3563, 46.9031)
  line L192 (118.6563, 34.9031) -> (118.5563, 34.9031)
  line L193 (118.8563, 35.2031) -> (118.8563, 35.1031)
  line L194 (119.3563, 35.4031) -> (119.0563, 35.4031)
  line L195 (119.8563, 34.9031) -> (119.8563, 32.9531)
  line L196 (118.3563, 34.7031) -> (118.3563, 28.4031)
  line L197 (138.3563, 34.7031) -> (138.3563, 28.4031)
  line L198 (136.8563, 34.9031) -> (136.8563, 32.9031)
  line L199 (137.8563, 35.2031) -> (137.8563, 35.1031)
  line L200 (138.0563, 34.9031) -> (138.1563, 34.9031)
  line L201 (137.3563, 35.4031) -> (137.6563, 35.4031)
  line L202 (138.0563, 41.9031) -> (138.1563, 41.9031)
  line L203 (137.8563, 41.6031) -> (137.8563, 41.7031)
  line L204 (137.3563, 41.4031) -> (137.6563, 41.4031)
  line L205 (136.8563, 41.9031) -> (136.8563, 43.9031)
  line L206 (138.3563, 42.1031) -> (138.3563, 46.9031)
  line L207 (124.6563, 48.4031) -> (119.8563, 48.4031)
  line L208 (124.8563, 46.9031) -> (122.8563, 46.9031)
  line L209 (125.3563, 47.4031) -> (125.3563, 47.7031)
  line L210 (125.1563, 47.9031) -> (125.0563, 47.9031)
  line L211 (124.8563, 48.1031) -> (124.8563, 48.2031)
  line L212 (132.0563, 48.4031) -> (136.8563, 48.4031)
  line L213 (131.8563, 46.9031) -> (133.8563, 46.9031)
  line L214 (131.5563, 47.9031) -> (131.6563, 47.9031)
  line L215 (131.8563, 48.1031) -> (131.8563, 48.2031)
  line L216 (131.3563, 47.4031) -> (131.3563, 47.7031)
  line L217 (130.8016, 37.1449) -> (131.304, 36.5161)
  line L218 (129.6145, 35.9578) -> (130.2434, 35.4554)
  line L219 (127.0981, 35.9578) -> (126.4693, 35.4554)
  line L220 (125.911, 37.1449) -> (125.4086, 36.5161)
  line L221 (125.911, 39.6613) -> (125.4086, 40.2902)
  line L222 (127.0981, 40.8484) -> (126.4693, 41.3508)
  line L223 (131.9422, 43.0496) -> (134.2099, 45.3173)
  line L224 (133.0028, 41.9889) -> (135.2705, 44.2567)
  line L225 (132.8563, 41.6353) -> (132.8563, 39.3567)
  line L226 (132.8295, 39.2567) -> (132.3944, 38.5031)
  line L227 (132.8295, 37.5495) -> (132.3944, 38.3031)
  line L228 (132.8563, 35.1709) -> (132.8563, 37.4495)
  line L229 (135.6241, 44.4031) -> (136.3563, 44.4031)
  line L230 (135.6241, 32.4031) -> (136.3563, 32.4031)
  line L231 (130.8016, 39.6613) -> (131.304, 40.2902)
  line L232 (133.0028, 34.8173) -> (135.2705, 32.5496)
  line L233 (131.5886, 33.9031) -> (129.3099, 33.9031)
  line L234 (129.2099, 33.9299) -> (128.4563, 34.365)
  line L235 (127.5027, 33.9299) -> (128.2563, 34.365)
  line L236 (125.1241, 33.9031) -> (127.4027, 33.9031)
  line L237 (131.9421, 33.7567) -> (134.6492, 31.0496)
  line L238 (124.7705, 33.7567) -> (122.0634, 31.0496)
  line L239 (123.8563, 35.1709) -> (123.8563, 37.4495)
  line L240 (123.8831, 37.5495) -> (124.3182, 38.3031)
  line L241 (123.8831, 39.2567) -> (124.3182, 38.5031)
  line L242 (123.8563, 41.6353) -> (123.8563, 39.3567)
  line L243 (121.1386, 32.4531) -> (120.3563, 32.4531)
  line L244 (121.0386, 44.4531) -> (120.3563, 44.4531)
  line L245 (123.7099, 34.8173) -> (121.4921, 32.5996)
  line L246 (123.7099, 41.9889) -> (121.3921, 44.3067)
  line L247 (129.6145, 40.8484) -> (130.2434, 41.3508)
  line L248 (124.7704, 43.0496) -> (122.5028, 45.3173)
  line L249 (134.3563, 45.6709) -> (134.3563, 46.4031)
  line L250 (122.3563, 45.6709) -> (122.3563, 46.4031)
  line L251 (131.5886, 42.9032) -> (129.31, 42.9032)
  line L252 (129.21, 42.8764) -> (128.4563, 42.4412)
  line L253 (127.5026, 42.8764) -> (128.2563, 42.4412)
  line L254 (125.124, 42.9032) -> (127.4026, 42.9032)
  line L255 (125.1241, 13.9031) -> (127.4027, 13.9031)
  line L256 (127.5027, 13.9299) -> (128.2563, 14.365)
  line L257 (129.2099, 13.9299) -> (128.4563, 14.365)
  line L258 (131.5885, 13.9031) -> (129.3099, 13.9031)
  line L259 (122.3563, 11.1353) -> (122.3563, 10.4031)
  line L260 (134.3563, 11.1353) -> (134.3563, 10.4031)
  line L261 (124.7705, 13.7567) -> (122.5028, 11.4889)
  line L262 (129.6145, 15.9578) -> (130.2434, 15.4554)
  line L263 (123.7099, 14.8173) -> (121.4421, 12.5496)
  line L264 (123.7099, 21.9889) -> (121.4421, 24.2567)
  line L265 (121.0885, 12.4031) -> (120.3563, 12.4031)
  line L266 (121.0886, 24.4031) -> (120.3563, 24.4031)
  line L267 (123.8563, 15.1709) -> (123.8563, 17.4495)
  line L268 (123.8831, 17.5495) -> (124.3182, 18.3031)
  line L269 (123.8831, 19.2567) -> (124.3182, 18.5031)
  line L270 (123.8563, 21.6353) -> (123.8563, 19.3567)
  line L271 (124.7703, 23.0497) -> (122.0634, 25.7567)
  line L272 (131.9423, 23.0497) -> (134.6492, 25.7567)
  line L273 (125.1239, 22.9032) -> (127.4025, 22.9032)
  arc A204 (129.2099, 33.9299) -> (129.3099, 33.9031) centre (129.3099, 34.1031) ccw
  arc A205 (125.1241, 33.9031) -> (124.7705, 33.7567) centre (125.1241, 33.4031) ccw
  arc A206 (131.9421, 33.7567) -> (131.5886, 33.9031) centre (131.5886, 33.4031) ccw
  arc A207 (124.3182, 38.3031) -> (124.3182, 38.5031) centre (124.145, 38.4031) ccw
  arc A208 (123.8563, 39.3567) -> (123.8831, 39.2567) centre (124.0563, 39.3567) ccw
  arc A209 (123.8831, 37.5495) -> (123.8563, 37.4495) centre (124.0563, 37.4495) ccw
  arc A210 (121.3921, 44.3067) -> (121.0386, 44.4531) centre (121.0386, 43.9531) ccw
  arc A211 (123.8563, 41.6353) -> (123.7099, 41.9889) centre (123.3563, 41.6353) ccw
  arc A212 (123.7099, 34.8173) -> (123.8563, 35.1709) centre (123.3563, 35.1709) ccw
  arc A213 (121.1386, 32.4531) -> (121.4921, 32.5996) centre (121.1386, 32.9531) ccw
  arc A214 (122.3563, 45.6709) -> (122.5028, 45.3173) centre (122.8563, 45.6709) ccw
  arc A215 (124.7704, 43.0496) -> (125.124, 42.9032) centre (125.124, 43.4032) ccw
  arc A216 (131.5886, 42.9032) -> (131.9422, 43.0496) centre (131.5886, 43.4032) ccw
  arc A217 (134.2099, 45.3173) -> (134.3563, 45.6709) centre (133.8563, 45.6709) ccw
  arc A218 (136.8563, 43.9031) -> (136.3563, 44.4031) centre (136.3563, 43.9031) ccw
  arc A219 (138.3563, 46.9031) -> (136.8563, 48.4031) centre (136.8563, 46.9031) ccw
  arc A220 (136.3563, 32.4031) -> (136.8563, 32.9031) centre (136.3563, 32.9031) ccw
  arc A221 (119.8563, 32.9531) -> (120.3563, 32.4531) centre (120.3563, 32.9531) ccw
  arc A222 (120.3563, 44.4531) -> (119.8563, 43.9531) centre (120.3563, 43.9531) ccw
  arc A223 (134.3563, 46.4031) -> (133.8563, 46.9031) centre (133.8563, 46.4031) ccw
  arc A224 (119.8563, 48.4031) -> (118.3563, 46.9031) centre (119.8563, 46.9031) ccw
  arc A225 (122.8563, 46.9031) -> (122.3563, 46.4031) centre (122.8563, 46.4031) ccw
  arc A226 (127.5026, 42.8764) -> (127.4026, 42.9032) centre (127.4026, 42.7032) ccw
  arc A227 (129.31, 42.9032) -> (129.21, 42.8764) centre (129.31, 42.7032) ccw
  arc A228 (128.2563, 42.4412) -> (128.4563, 42.4412) centre (128.3563, 42.6144) ccw
  arc A229 (129.6145, 40.8484) -> (127.0981, 40.8484) centre (128.3563, 38.4031) ccw
  arc A230 (127.0981, 15.9578) -> (129.6145, 15.9578) centre (128.3563, 18.4031) ccw
  arc A231 (128.4563, 14.365) -> (128.2563, 14.365) centre (128.3563, 14.1918) ccw
  arc A232 (129.2099, 13.9299) -> (129.3099, 13.9031) centre (129.3099, 14.1031) ccw
  arc A233 (127.4027, 13.9031) -> (127.5027, 13.9299) centre (127.4027, 14.1031) ccw
  arc A234 (122.3563, 10.4031) -> (122.8563, 9.9031) centre (122.8563, 10.4031) ccw
  arc A235 (118.3563, 9.9031) -> (119.8563, 8.4031) centre (119.8563, 9.9031) ccw
  arc A236 (133.8563, 9.9031) -> (134.3563, 10.4031) centre (133.8563, 10.4031) ccw
  arc A237 (119.8563, 12.9031) -> (120.3563, 12.4031) centre (120.3563, 12.9031) ccw
  arc A238 (120.3563, 24.4031) -> (119.8563, 23.9031) centre (120.3563, 23.9031) ccw
  arc A239 (136.8563, 23.9031) -> (136.3563, 24.4031) centre (136.3563, 23.9031) ccw
  arc A240 (136.8563, 8.4031) -> (138.3563, 9.9031) centre (136.8563, 9.9031) ccw
  arc A241 (136.3563, 12.4031) -> (136.8563, 12.9031) centre (136.3563, 12.9031) ccw
  arc A242 (134.3563, 11.1353) -> (134.2099, 11.4889) centre (133.8563, 11.1353) ccw
  arc A243 (131.9421, 13.7567) -> (131.5885, 13.9031) centre (131.5885, 13.4031) ccw
  arc A244 (125.1241, 13.9031) -> (124.7705, 13.7567) centre (125.1241, 13.4031) ccw
  arc A245 (122.5028, 11.4889) -> (122.3563, 11.1353) centre (122.8563, 11.1353) ccw
  arc A246 (121.4421, 24.2567) -> (121.0886, 24.4031) centre (121.0886, 23.9031) ccw
  arc A247 (123.8563, 21.6353) -> (123.7099, 21.9889) centre (123.3563, 21.6353) ccw
  arc A248 (123.7099, 14.8173) -> (123.8563, 15.1709) centre (123.3563, 15.1709) ccw
  arc A249 (121.0885, 12.4031) -> (121.4421, 12.5496) centre (121.0885, 12.9031) ccw
  arc A250 (123.8563, 19.3567) -> (123.8831, 19.2567) centre (124.0563, 19.3567) ccw
  arc A251 (123.8831, 17.5495) -> (123.8563, 17.4495) centre (124.0563, 17.4495) ccw
  arc A252 (124.3182, 18.3031) -> (124.3182, 18.5031) centre (124.145, 18.4031) ccw
  arc A253 (131.5887, 22.9032) -> (131.9423, 23.0497) centre (131.5887, 23.4032) ccw
  arc A254 (124.7703, 23.0497) -> (125.1239, 22.9032) centre (125.1239, 23.4032) ccw
  arc A255 (129.3101, 22.9032) -> (129.2101, 22.8764) centre (129.3101, 22.7032) ccw
  arc A256 (127.5025, 22.8764) -> (127.4025, 22.9032) centre (127.4025, 22.7032) ccw
  arc A257 (128.2563, 22.4412) -> (128.4563, 22.4412) centre (128.3563, 22.6144) ccw
  arc A258 (135.2705, 12.5496) -> (135.6241, 12.4031) centre (135.6241, 12.9031) ccw
  arc A259 (132.8563, 15.1709) -> (133.0028, 14.8173) centre (133.3563, 15.1709) ccw
  arc A260 (133.0028, 21.9889) -> (132.8563, 21.6353) centre (133.3563, 21.6353) ccw
  arc A261 (135.6241, 24.4031) -> (135.2705, 24.2567) centre (135.6241, 23.9031) ccw
  arc A262 (132.8563, 17.4495) -> (132.8295, 17.5495) centre (132.6563, 17.4495) ccw
  arc A263 (132.8295, 19.2567) -> (132.8563, 19.3567) centre (132.6563, 19.3567) ccw
  arc A264 (132.3944, 18.5031) -> (132.3944, 18.3031) centre (132.5676, 18.4031) ccw
  arc A265 (130.2434, 15.4554) -> (131.304, 16.5161) centre (128.3563, 18.4031) ccw
  arc A266 (125.4086, 16.5161) -> (126.4693, 15.4554) centre (128.3563, 18.4031) ccw
  arc A267 (126.4693, 21.3508) -> (125.4086, 20.2902) centre (128.3563, 18.4031) ccw
  arc A268 (131.304, 20.2902) -> (130.2434, 21.3508) centre (128.3563, 18.4031) ccw
  arc A269 (125.911, 19.6613) -> (125.911, 17.1449) centre (128.3563, 18.4031) ccw
  arc A270 (129.6145, 20.8484) -> (127.0981, 20.8484) centre (128.3563, 18.4031) ccw
  arc A271 (130.8016, 17.1449) -> (130.8016, 19.6613) centre (128.3563, 18.4031) ccw
  arc A272 (121.7099, 30.9031) -> (122.0634, 31.0496) centre (121.7099, 31.4031) ccw
  arc A273 (120.3563, 30.9031) -> (119.8563, 30.4031) centre (120.3563, 30.4031) ccw
  arc A274 (119.8563, 26.4031) -> (120.3563, 25.9031) centre (120.3563, 26.4031) ccw
  arc A275 (122.0634, 25.7567) -> (121.7099, 25.9031) centre (121.7099, 25.4031) ccw
  arc A276 (134.6492, 31.0496) -> (135.0028, 30.9031) centre (135.0028, 31.4031) ccw
  arc A277 (136.8563, 30.4031) -> (136.3563, 30.9031) centre (136.3563, 30.4031) ccw
  arc A278 (136.3563, 25.9031) -> (136.8563, 26.4031) centre (136.3563, 26.4031) ccw